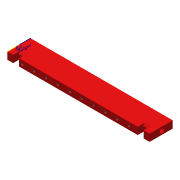
# Autodesk Inventor part: OuterOlfactometerChannel
Saved by Autodesk Inventor 2016 (Build 200138000, 138)
## iProperties
Created: 2011-11-24
Part Number: OuterOlfactometerChannel
Document SubType Name: Modeling
Designer: Neef
Density: 1.541 g/cm^3
Material: PET Plastic
Mass: 454.108 g
Surface Area: 238.698 cm^2
Volume: 56.2015 cm^3
Appearance: COLOUR1
Author: Neef
Autodesk Inventor part; units mm, degrees
ref_plane "YZ Plane" through (0, 0, 0) normal (1, 0, 0) x (0, 1, 0)
ref_plane "XZ Plane" through (0, 0, 0) normal (0, 1, 0) x (-1, 0, 0)
ref_plane "XY Plane" through (0, 0, 0) normal (0, 0, 1) x (1, 0, 0)
sketch "Skizze1" plane through (0, 0, 0) normal (0, 0, 1) x (1, 0, 0)
  line L0 (-120, 19.5) -> (120, 19.5)
  line L1 (120, 19.5) -> (120, -19.5)
  line L2 (120, -19.5) -> (-120, -19.5)
  line L3 (-120, -19.5) -> (-120, 19.5)
  line L4 (0, 27.3) -> (0, -27.3) projected
  line L5 (-168, 0) -> (168, 0) projected
  point P0 (0, 19.5)
  point P1 (120, 0)
  dimension "d0" = 39
  dimension "d1" = 240
  constraints: 8 end point, 2 midpoint, 2 parallel, 2 point on line, 1 horizontal, 1 perpendicular
  measures "d0" distance of L0.end L1.end
  measures "d1" distance of L0.start L0.end
extrude "Extrusion1" add sketch "Skizze1" along normal blind 12
sketch "Skizze6" plane through (0, 0, 0) normal (0, 0, -1) x (-1, 0, 0)
  line L0 (-120, -19.5) -> (120, -19.5) projected
  line L1 (120, -19.5) -> (120, 19.5) projected
  point P0 (95, -5.7)
  point P1 (95, -0.7)
  dimension "d77" = 25
  dimension "d79" = 18.8
  dimension "d80" = 13.8
  constraints: 1 vertical alignment
  measures "d77" distance from line of L1 point (95, -5.7)
  measures "d79" distance from line of L0 point (95, -0.7)
  measures "d80" distance from line of L0 point (95, -5.7)
hole "Bohrung7" at (-95, -5.7, 0) at (-95, -0.7, 0) direction (0, 0, 1) diameter 1.2 depth 6 tip angle 118
sketch "Skizze7" plane through (0, 0, 0) normal (0, 0, -1) x (-1, 0, 0)
  circle A0 centre (95, -5.7) radius 0.6 projected
  line L0 (-120, -19.5) -> (120, -19.5) projected
  point P0 (91.75, -4)
  point P1 (98.25, -4)
  dimension "d88" = 15.5
  dimension "d89" = 15.5
  dimension "d90" = 3.25
  dimension "d91" = 3.25
  measures "d88" distance from line of L0 point (98.25, -4)
  measures "d89" distance from line of L0 point (91.75, -4)
  measures "d90" horizontal distance of A0.centre point (98.25, -4)
  measures "d91" horizontal distance of A0.centre point (91.75, -4)
hole "Bohrung8" at (-91.75, -4, 0) at (-98.25, -4, 0) direction (0, 0, 1) diameter 1.221 depth 7 tip angle 118 thread size "M1.6x0.35" class "6H" standard "ISO Metric profile"
hole "Bohrung9" at (-95, -19.5, 6) direction (0, 1, 0) diameter 2 depth 14 tip angle 118
hole "Bohrung10" at (-95, -19.5, 6) direction (0, 1, 0) diameter 4.134 depth 7 tip angle 118 thread size "M5x0.8" class "6H" standard "ISO Metric profile"
pattern_linear "Rechteckige Anordnung3" count 10 spacing 20 along (1, 0, 0) of "Bohrung10", "Bohrung9", "Bohrung8", "Bohrung7"
sketch "Skizze19" plane through (0, 0, 12) normal (0, 0, 1) x (1, 0, 0)
  line L0 (120, -19.5) -> (-120, -19.5) projected
  line L1 (100, -19.5) -> (110, -19.5)
  line L2 (110, -19.5) -> (110, -10.5)
  line L3 (110, -10.5) -> (100, -10.5)
  line L4 (100, -10.5) -> (100, -19.5)
  line L5 (120, 19.5) -> (120, -19.5) projected
  line L6 (-120, 19.5) -> (120, 19.5) projected
  line L7 (0, 19.5) -> (0, -19.5)
  line L8 (-100, -19.5) -> (-110, -19.5)
  line L9 (-110, -19.5) -> (-110, -10.5)
  line L10 (-110, -10.5) -> (-100, -10.5)
  line L11 (-100, -10.5) -> (-100, -19.5)
  point P0 (0, 0)
  dimension "d319" = 10
  dimension "d320" = 10
  dimension "d321" = 9
  constraints: 18 end point, 4 symmetric about line, 2 midpoint, 2 parallel, 1 horizontal, 1 perpendicular, 1 point on line
  measures "d319" distance between parallel lines of L5 L2
  measures "d320" distance between parallel lines of L2 L4
  measures "d321" distance of L1.end L2.end
extrude "Extrusion6" cut sketch "Skizze19" against normal through all contours L0 L9 L10 L11 | L0 L4 L3 L2
chamfer "Fase2" distance 3 angle 45 4 edges at (105, -10.5, 12) (105, -10.5, 0) (-105, -10.5, 12) (-105, -10.5, 0)
sketch "Sketch21" plane through (120, -19.5, 0) normal (1, 0, 0) x (0, 0, -1)
  line L0 (0, 0) -> (0, 39) projected
  line L1 (0, 39) -> (-6, 39)
  line L2 (-6, 39) -> (-6, 21)
  line L3 (-6, 21) -> (0, 21)
  line L4 (0, 21) -> (0, 39)
  circle A0 centre (-6, 21) radius 4
  point P0 (0, 19.5)
  dimension "d341" = 6
  dimension "d342" = 18
  dimension "d343" = 8
  constraints: 8 end point, 2 parallel, 1 centre point, 1 coincident, 1 horizontal, 1 perpendicular
  measures "d341" distance of L3.end L2.end
  measures "d342" distance of L2.end L1.end
  measures "d343" diameter of A0
hole "Hole31" at (120, 1.5, 6) direction (-1, 0, 0) diameter 8 depth 220 tip angle 118
equation "\"d89\" = d88"
equation "\"d91\" = d90"
equation "\"d320\" = d319"
